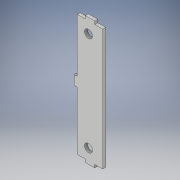
# Autodesk Inventor part: 1-8inch_Side1_2-Parts
Saved by Autodesk Inventor 2018 (Build 220112000, 112)
## iProperties
Created: 2018-01-31
Part Number: 1-8inch_Side1_2-Parts
Material: Generic
Document SubType Name: Modeling
Designer: lopezcha
Density: 1 g/cm^3
Appearance: Default
Author: lopezcha
Autodesk Inventor part; units mm, degrees
ref_plane "YZ Plane" through (0, 0, 0) normal (1, 0, 0) x (0, 1, 0)
ref_plane "XZ Plane" through (0, 0, 0) normal (0, 1, 0) x (-1, 0, 0)
ref_plane "XY Plane" through (0, 0, 0) normal (0, 0, 1) x (1, 0, 0)
sketch "Sketch1" plane through (0, 0, 0) normal (0, 0, 1) x (1, 0, 0)
  line L0 (3, 5) -> (3, 61.825)
  line L1 (11.5, 61.825) -> (11.5, 65)
  line L2 (11.5, 65) -> (21.5, 65)
  line L3 (21.5, 65) -> (21.5, 61.825)
  line L4 (30, 61.825) -> (30, -66.825)
  line L5 (21.5, -66.825) -> (21.5, -70)
  line L6 (21.5, -70) -> (11.5, -70)
  line L7 (11.5, -70) -> (11.5, -67)
  line L8 (3, -66.825) -> (3, -5)
  line L9 (3, -5) -> (0, -5)
  line L10 (0, 5) -> (3, 5)
  circle A0 centre (15, -55) radius 4.25
  circle A1 centre (15, 50) radius 4.25
  line L11 (3, 5) -> (3, 61.825)
  line L12 (11.5, 61.825) -> (11.5, 65)
  line L13 (11.5, 65) -> (21.5, 65)
  line L14 (21.5, 65) -> (21.5, 61.825)
  line L15 (30, 61.825) -> (30, -66.825)
  line L16 (21.5, -66.825) -> (21.5, -70)
  line L17 (21.5, -70) -> (11.5, -70)
  line L18 (11.5, -70) -> (11.5, -67)
  line L19 (3, -66.825) -> (3, -5)
  line L20 (3, -5) -> (0, -5)
  line L21 (0, 5) -> (3, 5)
  circle A2 centre (15, -55) radius 4.25
  circle A3 centre (15, 50) radius 4.25
  line L22 (11.5, 65) -> (21.5, 65)
  line L23 (21.5, 65) -> (21.5, 61.825)
  line L24 (11.5, 61.825) -> (11.5, 65)
  line L25 (3, 61.825) -> (11.5, 61.825)
  line L26 (21.5, 61.825) -> (30, 61.825)
  line L27 (11.5, -70) -> (21.5, -70)
  line L28 (21.5, -70) -> (21.5, -66.825)
  line L29 (11.5, -67) -> (11.5, -70)
  line L30 (30, -66.825) -> (21.5, -66.825)
  line L31 (3, 5) -> (-0.175, 5)
  line L32 (-0.175, 5) -> (-0.175, -5)
  line L33 (-0.175, -5) -> (3, -5)
  line L34 (11.5, -70) -> (11.5, -66.825)
  line L35 (11.5, -66.825) -> (3, -66.825)
  point P0 (0, 0)
  dimension "d2" = 3.175
  dimension "d3" = 3.175
  dimension "d4" = 3.175
  dimension "d7" = 3.175
  constraints: 74 end point, 4 centre point, 4 perpendicular, 3 horizontal, 3 parallel, 1 point on line
  measures "d2" distance of L3.end L22.end
  measures "d3" distance of L5.start L27.end
  measures "d4" distance of L8.end L32.end
  measures "d7" distance of L6.end L34.end
extrude "Extrusion3" add sketch "Sketch1" along normal blind 3.175
body "Solid3"
